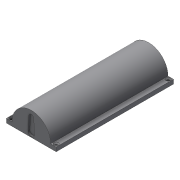
# Autodesk Inventor part: вал форточка
Saved by Autodesk Inventor 2021 (Build 250183000, 183)
## iProperties
Created: 2023-02-20
Part Number: вал форточка
Material: Типовые
Document SubType Name: Modeling
Designer: Tasya
Density: 1 g/cm^3
Appearance: По умолчанию
Author: Tasya
Autodesk Inventor part; units mm, degrees
ref_plane "YZ Plane" through (0, 0, 0) normal (1, 0, 0) x (0, 1, 0)
ref_plane "XZ Plane" through (0, 0, 0) normal (0, 1, 0) x (-1, 0, 0)
ref_plane "XY Plane" through (0, 0, 0) normal (0, 0, 1) x (1, 0, 0)
sketch "Эскиз1" plane through (0, 0, 0) normal (0, 0, 1) x (1, 0, 0)
  line L0 (0, 0) -> (-36, 0)
  line L1 (-36, 0) -> (-36, 6)
  line L2 (-36, 6) -> (-28, 6)
  arc A0 (0, 34) -> (-28, 6) centre (0, 6) ccw
  line L3 (0, 34) -> (0, 0) construction
  line L4 (-28, 6) -> (-28, 13.1241) construction
  circle A1 centre (0, 6) radius 4.75
  circle A2 centre (0, 25.75) radius 3.5
  line L5 (-3.493, 25.9715) -> (-4.7405, 6.3006)
  line L6 (3.493, 25.9715) -> (4.7405, 6.3006)
  line L7 (0, 0) -> (36, 0)
  line L8 (36, 0) -> (36, 6)
  line L9 (36, 6) -> (28, 6)
  arc A3 (28, 6) -> (0, 34) centre (0, 6) ccw
  line L10 (28, 6) -> (28, 13.1241) construction
  dimension "d0" = 8
  dimension "d1" = 6
  dimension "d2" = 28
  dimension "d3" = 7
  dimension "d4" = 9.5
  dimension "d5" = 19.75
  constraints: 22 end point, 8 point on circle, 5 tangent, 4 centre point, 4 symmetric about line, 2 perpendicular, 2 point on line, 2 vertical, 1 coincident, 1 horizontal, 1 other
  measures "d0" distance of L1.end L2.end
  measures "d1" distance of L0.end L1.end
  measures "d2" radius of A0
  measures "d3" diameter of A2
  measures "d4" diameter of A1
  measures "d5" distance of A0.centre A2.centre
extrude "Выдавливание1" add sketch "Эскиз1" along normal blind 170
sketch "Эскиз2" plane through (0, 0, 0) normal (0, 0, -1) x (-1, 0, 0)
  line L0 (-36, 6) -> (-28, 6) projected
  line L1 (-36, 0) -> (-36, 6) projected
  line L2 (36, 0) -> (-36, 0) projected
  line L3 (36, 6) -> (36, 0) projected
  line L4 (28, 6) -> (36, 6) projected
  arc A0 (28, 6) -> (-28, 6) centre (0, 6) ccw projected
  line L5 (-3.493, 25.9715) -> (-4.7405, 6.3006) projected
  arc A1 (3.493, 25.9715) -> (-3.493, 25.9715) centre (0, 25.75) ccw projected
  line L6 (4.7405, 6.3006) -> (3.493, 25.9715) projected
  arc A2 (-4.7405, 6.3006) -> (4.7405, 6.3006) centre (0, 6) ccw projected
  point P0 (0, 0)
extrude "Выдавливание2" add sketch "Эскиз2" against normal blind 167.5 contours A1 L6 A2 L5
sketch "Эскиз3" plane through (28, 6, 0) normal (0, 1, 0) x (1, 0, 0)
  line L0 (-64, 0) -> (8, 0) projected
  line L1 (8, 0) -> (8, -170) projected
  line L2 (-64, -170) -> (8, -170) projected
  line L3 (-64, 0) -> (-64, -170) projected
  line L4 (-28, 0) -> (-28, -85) construction
  line L5 (-28, -85) -> (14.415, -85) construction
  point P0 (-60, -166)
  point P1 (8, -85)
  point P2 (4, -166)
  point P3 (-60, -4)
  point P4 (4, -4)
  dimension "d10" = 4
  dimension "d11" = 4
  constraints: 4 end point, 3 symmetric about line, 1 midpoint, 1 perpendicular, 1 point on line, 1 vertical
  measures "d10" distance from line of L3 point (-60, -166)
  measures "d11" distance from line of L2 point (-60, -166)
hole "Отверстие1" at (-32, 6, 166) at (32, 6, 166) at (-32, 6, 4) at (32, 6, 4) direction (0, -1, 0) diameter 3.4 depth 6 countersink diameter 6.6 countersink angle 90 clearance for "с потайной головкой ГОСТ 12876-67" size "M3" standard "ГОСТ"
